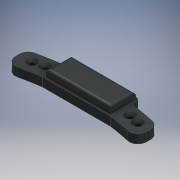
# Autodesk Inventor part: magnet
Saved by Autodesk Inventor 2018 (Build 220112000, 112)
## iProperties
Created: 2018-02-12
Part Number: magnet
Material: Iron, Gray
Document SubType Name: Modeling
Designer: JARVIS
Mass: 56.5194 g
Surface Area: 37.5365 cm^2
Volume: 7.90482 cm^3
Density: 7.15 g/cm^3
Appearance: Iron Gray
Author: JARVIS
Autodesk Inventor part; units mm, degrees
ref_plane "YZ Plane" through (0, 0, 0) normal (1, 0, 0) x (0, 1, 0)
ref_plane "XZ Plane" through (0, 0, 0) normal (0, 1, 0) x (-1, 0, 0)
ref_plane "XY Plane" through (0, 0, 0) normal (0, 0, 1) x (1, 0, 0)
sketch "Sketch1" plane through (0, 0, 0) normal (0, 0, 1) x (1, 0, 0)
  arc A0 (34.5919, 154.5766) -> (21.7257, 156.9029) centre (0, 0) ccw
  line L0 (38.5, 149.6973) -> (38.5, 147.1504)
  line L1 (-38.5, 147.1504) -> (-38.5, 149.6973)
  arc A1 (18.2237, 161.8774) -> (-18.2237, 161.8774) centre (0, 0) ccw
  line L2 (20, 159.8899) -> (20, 158.884)
  line L3 (-20, 158.884) -> (-20, 159.8899)
  arc A2 (-21.7257, 156.9029) -> (-34.5919, 154.5766) centre (0, 0) ccw
  arc A3 (32.3901, 142.2751) -> (20.1378, 144.5192) centre (0, 0) ccw
  arc A4 (-20.1378, 144.5192) -> (-32.3901, 142.2751) centre (0, 0) ccw
  line L4 (-19.8618, 144.5384) -> (19.8618, 144.5384)
  arc A5 (-38.5, 147.1504) -> (-32.3901, 142.2751) centre (-33.5, 147.1504) ccw
  arc A6 (-34.5919, 154.5766) -> (-38.5, 149.6973) centre (-33.5, 149.6973) ccw
  arc A7 (32.3901, 142.2751) -> (38.5, 147.1504) centre (33.5, 147.1504) ccw
  arc A8 (38.5, 149.6973) -> (34.5919, 154.5766) centre (33.5, 149.6973) ccw
  arc A9 (-21.7257, 156.9029) -> (-20, 158.884) centre (-22, 158.884) ccw
  arc A10 (20, 158.884) -> (21.7257, 156.9029) centre (22, 158.884) ccw
  arc A11 (20, 159.8899) -> (18.2237, 161.8774) centre (18, 159.8899) ccw
  arc A12 (-18.2237, 161.8774) -> (-20, 159.8899) centre (-18, 159.8899) ccw
  arc A13 (-19.8618, 144.5384) -> (-20.1378, 144.5192) centre (-19.8618, 142.5384) ccw
  arc A14 (20.1378, 144.5192) -> (19.8618, 144.5384) centre (19.8618, 142.5384) ccw
  point P0 (38.5, 140.7448)
  point P1 (38.5, 153.6499)
  point P2 (-38.5, 140.7448)
  point P3 (-38.5, 153.6499)
  point P4 (20, 161.6675)
  point P5 (20, 144.5384)
  point P6 (-20, 144.5384)
  point P7 (-20, 161.6675)
  point P8 (-20, 157.1322)
  point P9 (20, 157.1322)
  dimension "d5" = 77
  dimension "d6" = 38.5
  dimension "d9" = 5
  dimension "d10" = 2
  constraints: 41 point on circle, 20 tangent, 15 centre point, 10 end point, 10 point on line, 8 equal radius, 2 parallel, 1 coincident, 1 horizontal
  measures "d5" distance between parallel lines of L1 L0
  measures "d6" distance from line of point (0, 0) L1
  measures "d9" radius of A5
  measures "d10" radius of A9
extrude "Extrusion1" add sketch "Sketch1" along normal blind 5
sketch "Sketch2" plane through (0, 0, 5) normal (0, 0, 1) x (1, 0, 0)
  line L0 (-19, 145.5384) -> (19, 145.5384)
  line L1 (19, 145.5384) -> (19, 160.5384)
  line L2 (19, 160.5384) -> (-19, 160.5384)
  line L3 (-19, 160.5384) -> (-19, 145.5384)
  circle A0 centre (-31, 149.5384) radius 1.5
  circle A1 centre (-25, 151.0384) radius 1.5
  line L4 (-19.8618, 144.5384) -> (19.8618, 144.5384) projected
  point P0 (0, 0)
  point P1 (0, 145.5384)
  point P2 (0, 144.5384)
  dimension "d13" = 38
  dimension "d14" = 15
  dimension "d15" = 1
  dimension "d16" = 25
  dimension "d17" = 31
  dimension "d18" = 3
  dimension "d19" = 3
  dimension "d20" = 5
  dimension "d21" = 1.5
  constraints: 8 end point, 2 centre point, 2 midpoint, 2 parallel, 1 horizontal, 1 perpendicular, 1 vertical alignment
  measures "d13" distance of L1.end L2.end
  measures "d14" distance of L0.end L1.end
  measures "d15" distance between parallel lines of L0 L4
  measures "d16" horizontal distance of point (0, 144.538) A1.centre
  measures "d17" horizontal distance of point (0, 144.538) A0.centre
  measures "d18" diameter of A0
  measures "d19" diameter of A1
  measures "d20" vertical distance of point (0, 144.538) A0.centre
  measures "d21" vertical distance of A1.centre A0.centre
extrude "Extrusion2" add sketch "Sketch2" along normal blind 4 contours L3 L2 L1 L0
hole "Hole1" at (-31, 149.5384, 5) at (-25, 151.0384, 5) direction (0, 0, -1) diameter 3 end through all countersink diameter 6 countersink angle 90
mirror "Mirror1" about plane through (0, 0, 0) normal (1, 0, 0) of "Hole1"
fillet "Fillet1" radius 2 4 edges at (0, 160.5384, 9) (-19, 153.0384, 9) (0, 145.5384, 9) (19, 153.0384, 9)
equation "\"d6\" = 0.5 * d5"
equation "\"d19\" = d18"
body "Solid1"
